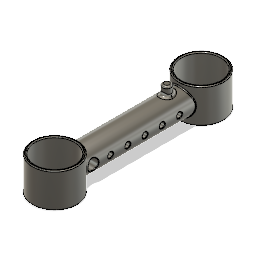
Electric Trombone Hand Piece v1 (Autodesk Fusion 360 design; units mm, degrees)
Autodesk Fusion 360 part; units mm, degrees
cylinder "CylinderPrimitive1" add diameter 26 height 20 placed x (1, 0, 0) y (0, 0, -1) z (0, 1, 0) at (10, 0, -10)
cylinder "CylinderPrimitive2" cut diameter 23 height -20 placed x (1, 0, 0) y (0, 0, -1) z (0, 1, 0) at (10, 20, -10)
cylinder "CylinderPrimitive3" add diameter 15 height 60 placed x (1, 0, 0) y (0, 1, 0) z (0, 0, 1) at (10, 10, 0)
cylinder "CylinderPrimitive4" cut diameter 23 height -20 placed x (1, 0, 0) y (0, 0, -1) z (0, 1, 0) at (10, 20, -10)
extrude "Extrude1" add 1 faces at (8.5574, 9.9186, 60) along direction (0, 0, 1) blind 10
cylinder "CylinderPrimitive5" add diameter 26 height 20 placed x (1, 0, 0) y (0, 0, -1) z (0, 1, 0) at (10, 0, 75)
cylinder "CylinderPrimitive6" cut diameter 23 height -20 placed x (1, 0, 0) y (0, 0, -1) z (0, 1, 0) at (10, 20, 75)
cylinder "CylinderPrimitive7" add diameter 5 height -10 placed x (1, 0, 0) y (0, 0, -1) z (0, 1, 0) at (10, 20, 10)
extrude "Extrude2" add 1 faces at (10.7914, 20, 10.9038) along direction (0, 1, 0) blind 4
cylinder "CylinderPrimitive8" cut diameter 3 height 100 placed x (0, 0, -1) y (0, 1, 0) z (1, 0, 0) at (0, 10, 10)
cylinder "CylinderPrimitive9" cut diameter 3 height 200 placed x (0, 0, -1) y (0, 1, 0) z (1, 0, 0) at (0, 10, 20)
cylinder "CylinderPrimitive10" cut diameter 3 height 200 placed x (0, 0, -1) y (0, 1, 0) z (1, 0, 0) at (0, 10, 30)
cylinder "CylinderPrimitive11" cut diameter 3 height 200 placed x (0, 0, -1) y (0, 1, 0) z (1, 0, 0) at (0, 10, 40)
cylinder "CylinderPrimitive12" cut diameter 3 height 200 placed x (0, 0, -1) y (0, 1, 0) z (1, 0, 0) at (0, 10, 50)
cylinder "CylinderPrimitive13" cut diameter 6 height 200 placed x (0, 0, -1) y (0, 1, 0) z (1, 0, 0) at (0, 10, 60)
fillet "Fillet1" radius 0.5 1 faces at (1.1063, 9.9273, -0.5183)
fillet "Fillet2" radius 0.5 1 faces at (11.145, 6.6667, -21.4429)
fillet "Fillet3" radius 0.5 1 faces at (0.966, 9.8292, 65.6519)
fillet "Fillet4" radius 0.5 1 faces at (11.145, 6.6667, 63.5571)
fillet "Fillet5" radius 0.25 1 faces at (7.5462, 8.5454, 57.3762)
fillet "Fillet6" radius 0.25 1 faces at (7.5016, 10.0839, 51.4977)
fillet "Fillet7" radius 0.25 1 faces at (7.5016, 10.0839, 41.4977)
fillet "Fillet8" radius 0.25 1 faces at (7.5016, 10.0839, 31.4977)
fillet "Fillet9" radius 0.25 1 faces at (7.5016, 10.0839, 21.4977)
fillet "Fillet10" radius 0.25 1 faces at (7.5016, 10.0839, 11.4977)
fillet "Fillet11" radius 2 1 edges at (7.5, 17.0711, 10)
extrude "Extrude3" cut 1 faces at (9.4804, 24, 9.5179) along direction (0, -1, 0) blind 1.5
fillet "Fillet12" radius 1 1 edges at (9.096, 22.5, 12.3308)
